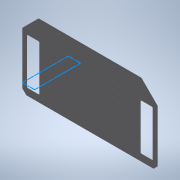
# Autodesk Inventor part: PlanchaBaseInferior
Saved by Autodesk Inventor 2022.1 (Build 261234000, 234)
## iProperties
Created: 2021-09-22
Part Number: PlanchaBaseInferior
Material: Steel, Mild, Welded
Document SubType Name: Sheet Metal
Designer: Andres
Density: 7.85 g/cm^3
Sheet Metal Rule: Por defecto_mm
Appearance: Weld - Steel Mild
Author: Andres
Autodesk Inventor part; units mm, degrees
ref_plane "YZ Plane" through (0, 0, 0) normal (1, 0, 0) x (0, 1, 0)
ref_plane "XZ Plane" through (0, 0, 0) normal (0, 1, 0) x (-1, 0, 0)
ref_plane "XY Plane" through (0, 0, 0) normal (0, 0, 1) x (1, 0, 0)
sketch "Sketch1" plane through (0, 0, 0) normal (0, 0, 1) x (1, 0, 0)
  line L0 (126.4853, -346.4853) -> (-16.5442, -346.4853) construction
  line L1 (-16.5442, -346.4853) -> (-29.5147, -333.5147) construction
  line L2 (-29.5147, -333.5147) -> (-29.5147, -13.4558) construction
  line L3 (-29.5147, -13.4558) -> (63.4558, 79.5147) construction
  line L4 (63.4558, 79.5147) -> (126.4853, 79.5147) construction
  line L5 (750.4853, 79.5147) -> (813.5147, 79.5147) construction
  line L6 (570.4853, 79.5147) -> (726.4853, 79.5147) construction
  line L7 (150.4853, 79.5147) -> (306.4853, 79.5147) construction
  line L8 (330.4853, 79.5147) -> (546.4853, 79.5147) construction
  line L9 (813.5147, 79.5147) -> (906.4853, -13.4558) construction
  line L10 (906.4853, -13.4558) -> (906.4853, -333.5147) construction
  line L11 (906.4853, -333.5147) -> (893.5147, -346.4853) construction
  line L12 (893.5147, -346.4853) -> (750.4853, -346.4853) construction
  line L13 (903.4558, -370.4853) -> (750.4853, -370.4853) construction
  line L14 (930.4853, -343.4558) -> (903.4558, -370.4853) construction
  line L15 (930.4853, -3.5147) -> (930.4853, -343.4558) construction
  line L16 (823.4558, 103.5147) -> (930.4853, -3.5147) construction
  line L17 (53.5147, 103.5147) -> (823.4558, 103.5147) construction
  line L18 (-53.5147, -3.5147) -> (53.5147, 103.5147) construction
  line L19 (-53.5147, -343.4558) -> (-53.5147, -3.5147) construction
  line L20 (-26.4853, -370.4853) -> (-53.5147, -343.4558) construction
  line L21 (126.4853, -370.4853) -> (-26.4853, -370.4853) construction
  line L22 (726.4853, -370.4853) -> (570.4853, -370.4853) construction
  line L23 (726.4853, -346.4853) -> (570.4853, -346.4853) construction
  line L24 (726.4853, -346.4853) -> (570.4853, -346.4853) construction
  line L25 (726.4853, -370.4853) -> (570.4853, -370.4853) construction
  line L26 (726.4853, -370.4853) -> (570.4853, -370.4853) construction
  line L27 (726.4853, -346.4853) -> (570.4853, -346.4853) construction
  line L28 (930.4853, -3.5147) -> (930.4853, -343.4558)
  line L29 (903.4558, -370.4853) -> (-26.4853, -370.4853)
  line L30 (-26.4853, -370.4853) -> (-53.5147, -343.4558)
  line L31 (-53.5147, -343.4558) -> (-53.5147, -3.5147)
  line L32 (-53.5147, -3.5147) -> (53.5147, 103.5147)
  line L33 (53.5147, 103.5147) -> (823.4558, 103.5147)
  line L34 (823.4558, 103.5147) -> (930.4853, -3.5147)
  line L35 (930.4853, -343.4558) -> (903.4558, -370.4853)
  line L36 (726.4853, -370.4853) -> (726.4853, -346.4853)
  line L37 (570.4853, -346.4853) -> (570.4853, -370.4853)
  line L38 (126.4853, -370.4853) -> (126.4853, -346.4853)
  line L39 (126.4853, 79.5147) -> (126.4853, 91.5147)
  line L40 (126.4853, 91.5147) -> (150.4853, 91.5147)
  line L41 (150.4853, 79.5147) -> (150.4853, 91.5147)
  line L42 (306.4853, 91.5147) -> (306.4853, 79.5147)
  line L43 (306.4853, 91.5147) -> (330.4853, 91.5147)
  line L44 (330.4853, 91.5147) -> (330.4853, 79.5147)
  line L45 (546.4853, 91.5147) -> (546.4853, 79.5147)
  line L46 (546.4853, 91.5147) -> (570.4853, 91.5147)
  line L47 (570.4853, 91.5147) -> (570.4853, 79.5147)
  line L48 (726.4853, 79.5147) -> (726.4853, 91.5147)
  line L49 (726.4853, 91.5147) -> (750.4853, 91.5147)
  line L50 (750.4853, 79.5147) -> (750.4853, 91.5147)
  line L51 (750.4853, -370.4853) -> (750.4853, -346.4853)
  line L52 (726.4853, -370.4853) -> (726.4853, -346.4853)
  line L53 (570.4853, -346.4853) -> (570.4853, -370.4853)
  line L54 (726.4853, -370.4853) -> (726.4853, -346.4853)
  line L55 (570.4853, -346.4853) -> (570.4853, -370.4853)
  point P0 (0, 0)
extrude "Plate1" add sketch "Sketch1" along normal blind 0.5
sketch "Sketch2" plane through (0, 0, 0.5) normal (0, 0, 1) x (1, 0, 0)
  line L0 (78.4853, -25.4853) -> (-21.5147, -25.4853)
  line L1 (-21.5147, -25.4853) -> (-21.5147, -325.4853)
  line L2 (-21.5147, -325.4853) -> (78.4853, -325.4853)
  line L3 (78.4853, -325.4853) -> (78.4853, -25.4853)
  line L4 (78.4853, -25.4853) -> (-21.5147, -325.4853) construction
  line L5 (-21.5147, -25.4853) -> (78.4853, -325.4853) construction
  line L6 (119.5571, -370.4853) -> (-26.4853, -370.4853) projected
  line L7 (-26.4853, -370.4853) -> (-53.5147, -343.4558) projected
  line L8 (-53.5147, -343.4558) -> (-53.5147, -3.5147) projected
  line L9 (-53.5147, -3.5147) -> (53.5147, 103.5147) projected
  line L10 (53.5147, 103.5147) -> (823.4558, 103.5147) projected
  line L11 (823.4558, 103.5147) -> (930.4853, -3.5147) projected
  line L12 (930.4853, -3.5147) -> (930.4853, -343.4558) projected
  line L13 (930.4853, -343.4558) -> (903.4558, -370.4853) projected
  line L14 (903.4558, -370.4853) -> (757.4135, -370.4853) projected
  line L15 (893.5147, -346.4853) -> (757.4135, -346.4853) projected
  line L16 (906.4853, -333.5147) -> (893.5147, -346.4853) projected
  line L17 (906.4853, -13.4558) -> (906.4853, -333.5147) projected
  line L18 (813.5147, 79.5147) -> (906.4853, -13.4558) projected
  line L19 (757.4135, 79.5147) -> (813.5147, 79.5147) projected
  line L20 (577.4135, 79.5147) -> (719.5571, 79.5147) projected
  line L21 (337.4135, 79.5147) -> (539.5571, 79.5147) projected
  line L22 (63.4558, 79.5147) -> (119.5571, 79.5147) projected
  line L23 (157.4135, 79.5147) -> (299.5571, 79.5147) projected
  line L24 (-29.5147, -13.4558) -> (63.4558, 79.5147) projected
  line L25 (-29.5147, -333.5147) -> (-29.5147, -13.4558) projected
  line L26 (-16.5442, -346.4853) -> (-29.5147, -333.5147) projected
  line L27 (119.5571, -346.4853) -> (-16.5442, -346.4853) projected
  line L28 (438.4853, 188.8971) -> (438.4853, -449.5258) construction
  line L29 (798.4853, -25.4853) -> (898.4853, -25.4853)
  line L30 (898.4853, -25.4853) -> (898.4853, -325.4853)
  line L31 (898.4853, -325.4853) -> (798.4853, -325.4853)
  line L32 (798.4853, -325.4853) -> (798.4853, -25.4853)
  line L33 (798.4853, -25.4853) -> (898.4853, -325.4853) construction
  line L34 (898.4853, -25.4853) -> (798.4853, -325.4853) construction
  line L35 (119.5571, -346.4853) -> (119.5571, -370.4853) projected
  line L36 (757.4135, -370.4853) -> (757.4135, -346.4853) projected
  line L37 (757.4135, 79.5147) -> (757.4135, 91.5147) projected
  line L38 (757.4135, 91.5147) -> (719.5571, 91.5147) projected
  line L39 (719.5571, 91.5147) -> (719.5571, 79.5147) projected
  line L40 (577.4135, 79.5147) -> (577.4135, 91.5147) projected
  line L41 (577.4135, 91.5147) -> (539.5571, 91.5147) projected
  line L42 (539.5571, 91.5147) -> (539.5571, 79.5147) projected
  line L43 (337.4135, 79.5147) -> (337.4135, 91.5147) projected
  line L44 (337.4135, 91.5147) -> (299.5571, 91.5147) projected
  line L45 (299.5571, 91.5147) -> (299.5571, 79.5147) projected
  line L46 (157.4135, 79.5147) -> (157.4135, 91.5147) projected
  line L47 (157.4135, 91.5147) -> (119.5571, 91.5147) projected
  line L48 (119.5571, 91.5147) -> (119.5571, 79.5147) projected
  point P0 (0, 0)
  point P1 (28.4853, -175.4853)
  point P2 (438.4853, 79.5147)
  point P3 (848.4853, -175.4853)
  dimension "d1" = 100
  dimension "d2" = 300
  dimension "d4" = 410
  dimension "d5" = 255
  constraints: 26 end point, 5 midpoint, 5 symmetric about line, 2 parallel, 1 horizontal, 1 perpendicular, 1 vertical, 1 vertical alignment, 1 other
  measures "d1" distance between parallel lines of L1 L3
  measures "d2" distance between parallel lines of L2 L0
  measures "d4" distance from line of point (28.485, -175.485) L28
  measures "d5" vertical distance of point (438.485, 79.515) point (28.485, -175.485)
extrude "Cut1" cut sketch "Sketch2" against normal through all contours L3 L2 L1 L0 | L29 L30 L31 L32
fillet "Corner Round1" radius 6 8 edges at (78.4853, -25.4853, 0.25) (-21.5147, -25.4853, 0.25) (-21.5147, -325.4853, 0.25) (78.4853, -325.4853, 0.25) (898.4853, -25.4853, 0.25) (798.4853, -25.4853, 0.25) (898.4853, -325.4853, 0.25) (798.4853, -325.4853, 0.25)
equation "\"d6\" = Thickness"
equation "\"d0\" = Thickness"
equation "\"BendRadius\" = Thickness"
equation "\"BendReliefWidth\" = Thickness"
equation "\"BendReliefDepth\" = 0.5 * Thickness"
equation "\"CornerReliefSize\" = 4 * Thickness"
equation "\"MinimumRemnant\" = 2 * Thickness"
equation "\"TransitionRadius\" = BendRadius"
equation "\"JacobiRadiusSize\" = BendRadius"
equation "\"GapSize\" = Thickness"
equation "\"Thickness\" = 0.5"
body "Solid1"
